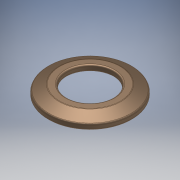
# Autodesk Inventor part: PODKŁADKA M6x11
Saved by Autodesk Inventor 2017 SP1 (Build 210196100, 196)
## iProperties
Created: 2021-02-09
Part Number: PODKŁADKA M6x11
Material: Stal
Document SubType Name: Modeling
Designer: Napoleon
Mass: 0.444742 g
Surface Area: 1.70094 cm^2
Volume: 0.0566551 cm^3
Density: 7.85 g/cm^3
Appearance: Anodowany - brązowy
Author: Napoleon
Autodesk Inventor part; units mm, degrees
ref_plane "YZ Plane" through (0, 0, 0) normal (1, 0, 0) x (0, 1, 0)
ref_plane "XZ Plane" through (0, 0, 0) normal (0, 1, 0) x (-1, 0, 0)
ref_plane "XY Plane" through (0, 0, 0) normal (0, 0, 1) x (1, 0, 0)
sketch "Szkic1" plane through (0, 0, 0) normal (0, 0, 1) x (1, 0, 0)
  circle A0 centre (0, 0) radius 3
  circle A1 centre (0, 0) radius 5.475
  dimension "d3" = 6
  dimension "d4" = 10.95
  constraints: 2 centre point, 2 coincident
  measures "d3" diameter of A0
  measures "d4" diameter of A1
extrude "Wyciągnięcie proste1" add sketch "Szkic1" along normal mid plane 1.4
chamfer "Faza1" distance 1.5 distance2 0.7 1 edges at (-5.475, 0, 0.7) measured on face at (4.597, -0.4368, 0.7)
chamfer "Faza2" distance 2.25 distance2 0.7 1 edges at (-3, 0, -0.7) measured on face at (4.597, -0.4368, -0.7)
fillet "Zaokrąglenie2" radius 0.2 8 edges at (-3, 0, -0.0005) (-3, 0, 0) (-5.2495, 0, -0.7) (-5.475, 0, -0.7) (-5.475, 0, 0) (-5.475, 0, 0.0005) (-3.9755, 0, 0.7) (-3, 0, 0.7)
